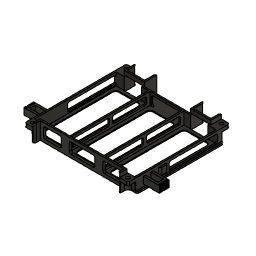
BatteryBase (Autodesk Fusion 360 design; units mm, degrees)
Autodesk Fusion 360 part; units mm, degrees
sketch "草图1" plane through (0, 0, 0) normal (0, 0, 1) x (1, 0, 0)
  line L0 (31, 31.5) -> (-31, 31.5)
  line L1 (-32, 30.5) -> (-32, -30.5)
  line L2 (-31, -31.5) -> (31, -31.5)
  line L3 (32, -30.5) -> (32, 30.5)
  line L4 (32, 31.5) -> (-32, -31.5) construction
  line L5 (-32, 31.5) -> (32, -31.5) construction
  arc A0 (-31, 31.5) -> (-32, 30.5) centre (-31, 30.5) ccw
  arc A1 (-32, -30.5) -> (-31, -31.5) centre (-31, -30.5) ccw
  arc A2 (31, -31.5) -> (32, -30.5) centre (31, -30.5) ccw
  arc A3 (32, 30.5) -> (31, 31.5) centre (31, 30.5) ccw
  dimension "d3" = 1
  dimension "d4" = 1
  dimension "d5" = 1
  dimension "d6" = 1
  dimension "d7" = 64
  dimension "d8" = 63
  constraint horizontal L0
  constraint perpendicular L0 L1
  constraint parallel L0 L2
  constraint parallel L1 L3
  constraint coincident L4 origin
  constraint coincident L5 origin
  constraint coincident L5.start L1
  constraint coincident L5.start L0
  constraint tangent L1 A0
  constraint tangent L0 A0
  constraint coincident L4.end L1
  constraint coincident L4.end L2
  constraint tangent L1 A1
  constraint tangent L2 A1
  constraint coincident L5.end L2
  constraint coincident L5.end L3
  constraint tangent L2 A2
  constraint tangent L3 A2
  constraint coincident L4.start L0
  constraint coincident L4.start L3
  constraint tangent L0 A3
  constraint tangent L3 A3
  measures "d3" radius of A0
  measures "d4" radius of A1
  measures "d5" radius of A2
  measures "d6" radius of A3
  measures "d7" distance of L1 L3
  measures "d8" distance of L0 L2
extrude "拉伸1" add sketch "草图1" along normal blind 10.6 makes body 1
sketch "草图2" plane through (0, 0, 10.6) normal (0, 0, 1) x (-1, 0, 0)
  arc A0 (-32, -30.5) -> (-31, -31.5) centre (-31, -30.5) ccw
  line L0 (-31, -31.5) -> (31, -31.5)
  arc A1 (31, -31.5) -> (32, -30.5) centre (31, -30.5) ccw
  line L1 (32, -30.5) -> (32, 30.5)
  arc A2 (32, 30.5) -> (31, 31.5) centre (31, 30.5) ccw
  line L2 (31, 31.5) -> (-31, 31.5)
  arc A3 (-31, 31.5) -> (-32, 30.5) centre (-31, 30.5) ccw
  line L3 (-32, 30.5) -> (-32, -30.5)
  line L4 (32.1, -24.5) -> (26.9, -24.5)
  line L5 (26.9, -24.5) -> (26.9, -31.5)
  line L6 (26.9, -31.5) -> (32.1, -31.5)
  line L7 (32.1, -31.5) -> (32.1, -24.5)
  line L8 (0, -35) -> (0, 35) construction
  line L9 (42, 0) -> (-42, 0) construction
  line L10 (-26.9, -24.5) -> (-26.9, -31.5)
  line L11 (-26.9, -31.5) -> (-32.1, -31.5)
  line L12 (-32.1, -24.5) -> (-26.9, -24.5)
  line L13 (-32.1, -31.5) -> (-32.1, -24.5)
  line L14 (26.9, 24.5) -> (26.9, 31.5)
  line L15 (26.9, 31.5) -> (32.1, 31.5)
  line L16 (32.1, 31.5) -> (32.1, 24.5)
  line L17 (32.1, 24.5) -> (26.9, 24.5)
  line L18 (-26.9, 31.5) -> (-32.1, 31.5)
  line L19 (-26.9, 24.5) -> (-26.9, 31.5)
  line L20 (-32.1, 24.5) -> (-26.9, 24.5)
  line L21 (-32.1, 31.5) -> (-32.1, 24.5)
  point P0 (-31, -30.5)
  point P1 (-31, -31.5)
  point P2 (31, 30.5)
  point P3 (31, 31.5)
  point P4 (-31, 30.5)
  point P5 (-31, 31.5)
  point P6 (-31, 30.5)
  point P7 (-31, 31.5)
  dimension "d11" = 26.9
  dimension "d12" = 5.2
  dimension "d13" = 7
  constraint horizontal L4
  constraint vertical L5
  constraint horizontal L6
  constraint vertical L7
  constraint coincident L0 L5.end
  constraint perpendicular L2 L8
  constraint perpendicular L3 L9
  constraint symmetric L0.end L8 P1
  constraint symmetric A1.centre L8 P0
  constraint symmetric L4.start L8 L12.start
  constraint symmetric L4.end L8 L10.start
  constraint symmetric L5.end L8 L10.end
  constraint symmetric L6.end L8 L11.end
  constraint symmetric L0.end L9 P3
  constraint symmetric A1.centre L9 P2
  constraint symmetric L4.start L9 L16.end
  constraint symmetric L4.end L9 L14.start
  constraint symmetric L5.end L9 L14.end
  constraint symmetric L6.end L9 L15.end
  constraint symmetric P1 L9 P7
  constraint symmetric P0 L9 P6
  constraint symmetric L9 P0 P6
  constraint symmetric L9 L11.end L18.end
  constraint symmetric L9 L10.end L18.start
  constraint symmetric L9 P1 P7
  constraint symmetric L9 L10.start L19.start
  constraint symmetric L9 L12.start L20.start
  measures "d11" distance of origin L5
  measures "d12" distance of L4.start L4.end
  measures "d13" distance of L4 L6
extrude "拉伸2" cut sketch "草图2" against normal blind 2.5 contours A0 L0 L3 L10 L11 L12 | A0 L3 L11 L12 L13 | A3 L3 L18 L20 L21 | L2 A3 L3 L18 L19 L20 | L0 A1 L1 L4 L5 L6 | A1 L1 L4 L6 L7 | L1 A2 L2 L14 L15 L17 | L1 A2 L15 L16 L17 bodies 1
sketch "草图3" plane through (0, 0, 10.6) normal (0, 0, 1) x (-1, 0, 0)
  line L0 (32, -25) -> (-32, -25)
  line L1 (-32, -25) -> (-32, 27)
  line L2 (-32, 27) -> (32, 27)
  line L3 (32, 27) -> (32, -25)
  dimension "d206" = 25
  dimension "d207" = 32
  dimension "d208" = 32
  dimension "d209" = 27
  constraint horizontal L0
  constraint vertical L1
  constraint horizontal L2
  constraint vertical L3
  measures "d206" distance of origin L0
  measures "d207" distance of origin L3
  measures "d208" distance of origin L1
  measures "d209" distance of origin L2
extrude "拉伸3" cut sketch "草图3" against normal blind 2.5 bodies 1
sketch "草图5" plane through (0, 0, 8.1) normal (0, 0, 1) x (-1, 0, 0)
  circle A0 centre (29.5, -29) radius 1.1
  line L0 (0, -32.9404) -> (0, 32.0596) construction
  line L1 (41.6677, 0) -> (-40.3323, 0) construction
  circle A1 centre (-29.5, -29) radius 1.1
  circle A2 centre (29.5, 29) radius 1.1
  circle A3 centre (-29.5, 29) radius 1.1
  arc A4 (-31, 31.5) -> (-32, 30.5) centre (-31, 30.5) ccw
  line L2 (-32, 30.5) -> (-32, -30.5)
  line L3 (-26.9, 27) -> (-26.9, 31.5)
  line L4 (-26.9, 31.5) -> (-31, 31.5)
  line L5 (32, -30.5) -> (32, 30.5)
  arc A5 (32, 30.5) -> (31, 31.5) centre (31, 30.5) ccw
  line L6 (26.9, 31.5) -> (26.9, 27)
  line L7 (-26.9, -25) -> (26.9, -25)
  line L8 (31, 31.5) -> (26.9, 31.5)
  line L9 (26.9, 27) -> (-26.9, 27)
  arc A6 (-32, -30.5) -> (-31, -31.5) centre (-31, -30.5) ccw
  line L10 (-31, -31.5) -> (-26.9, -31.5)
  line L11 (-26.9, -31.5) -> (-26.9, -25)
  line L12 (26.9, -25) -> (26.9, -31.5)
  line L13 (26.9, -31.5) -> (31, -31.5)
  arc A7 (31, -31.5) -> (32, -30.5) centre (31, -30.5) ccw
  line L14 (31, -31.5) -> (26.9, -31.5)
  line L15 (-26.9, -31.5) -> (-31, -31.5)
  dimension "d20" = 2.2
  dimension "d21" = 29.5
  constraint horizontal L1
  constraint symmetric A0 L0 A1
  constraint symmetric A0 L1 A2
  constraint symmetric L1 A1 A3
  constraint coincident origin L1
  measures "d20" diameter of A0
  measures "d21" distance of A0.centre L0
extrude "拉伸4" cut sketch "草图5" against normal blind 12 contours A0 | A1 | A2 | A3 bodies 1
sketch "草图6" plane through (0, 0, 8.1) normal (0, 0, 1) x (-1, 0, 0)
  line L0 (10, 26.5) -> (-10, 26.5)
  line L1 (-10, 26.5) -> (-10, -24.1)
  line L2 (-10, -24.1) -> (10, -24.1)
  line L3 (10, -24.1) -> (10, 26.5)
  line L4 (11, 26.5) -> (11, -24.1)
  line L5 (11, -24.1) -> (31, -24.1)
  line L6 (31, -24.1) -> (31, 26.5)
  line L7 (31, 26.5) -> (11, 26.5)
  line L8 (-11, -24.1) -> (-11, 26.5)
  line L9 (-31, -24.1) -> (-11, -24.1)
  line L10 (-31, 26.5) -> (-31, -24.1)
  line L11 (-11, 26.5) -> (-31, 26.5)
  point P0 (23, 0)
  dimension "d25" = 50.6
  dimension "d26" = 20
  dimension "d28" = 10
  dimension "d160" = 24.1
  dimension "d200" = 21
  dimension "d201" = 0
  dimension "d204" = -21
  dimension "d205" = 0
  constraint horizontal L0
  constraint vertical L1
  constraint horizontal L2
  constraint vertical L3
  measures "d25" distance of L0 L2
  measures "d26" distance of L1 L3
  measures "d28" distance of origin L3
  measures "d160" distance of origin L2
extrude "拉伸5" cut sketch "草图6" against normal blind 7.5 bodies 1
sketch "草图7" plane through (0, 0, 10.6) normal (0, 0, 1) x (-1, 0, 0)
  line L0 (14.2, -32.5) -> (-14.2, -32.5)
  line L1 (-14.2, -32.5) -> (-14.2, -25)
  line L2 (-14.2, -25) -> (14.2, -25)
  line L3 (14.2, -25) -> (14.2, -32.5)
  line L4 (-26.9, -31.5) -> (26.9, -31.5)
  dimension "d210" = 28.4
  dimension "d211" = 14.2
  dimension "d212" = 7.5
  dimension "d213" = 1
  constraint horizontal L0
  constraint vertical L1
  constraint horizontal L2
  constraint vertical L3
  measures "d210" distance of L0.start L0.end
  measures "d211" distance of origin L3
  measures "d212" distance of L0 L2
  measures "d213" distance of L0 L4
extrude "拉伸6" cut sketch "草图7" against normal blind 10 contours L1 L2 L3 L4 bodies 1
sketch "草图8" plane through (0, 0, 0) normal (0, 0, -1) x (1, 0, 0)
  circle A0 centre (29.5, -29) radius 1.1
  circle A1 centre (29.5, 29) radius 1.1
  circle A2 centre (-29.5, -29) radius 1.1
  circle A3 centre (-29.5, 29) radius 1.1
  arc A4 (31, -31.5) -> (32, -30.5) centre (31, -30.5) ccw
  line L0 (32, -30.5) -> (32, 30.5)
  arc A5 (32, 30.5) -> (31, 31.5) centre (31, 30.5) ccw
  line L1 (31, 31.5) -> (-31, 31.5)
  arc A6 (-31, 31.5) -> (-32, 30.5) centre (-31, 30.5) ccw
  line L2 (-32, 30.5) -> (-32, -30.5)
  arc A7 (-32, -30.5) -> (-31, -31.5) centre (-31, -30.5) ccw
  line L3 (-31, -31.5) -> (31, -31.5)
  line L4 (-27.25, -31.5) -> (-27.25, -29)
  arc A8 (-27.25, -29) -> (-29.5, -26.75) centre (-29.5, -29) ccw
  line L5 (-29.5, -26.75) -> (-32, -26.75)
  line L6 (-27.25, -31.5) -> (-32, -31.5)
  line L7 (-32, -31.5) -> (-32, -26.75)
  line L8 (0, 0) -> (0, -35.7706) construction
  line L9 (27.25, -31.5) -> (32, -31.5)
  line L10 (32, -31.5) -> (32, -26.75)
  circle A9 centre (29.5, -29) radius 1.1
  arc A10 (31, -31.5) -> (32, -30.5) centre (31, -30.5) ccw
  line L11 (27.25, -31.5) -> (27.25, -29)
  line L12 (29.5, -26.75) -> (32, -26.75)
  arc A11 (29.5, -26.75) -> (27.25, -29) centre (29.5, -29) ccw
  line L13 (0, 0) -> (-39, 0) construction
  arc A12 (27.25, 29) -> (29.5, 26.75) centre (29.5, 29) ccw
  line L14 (27.25, 31.5) -> (32, 31.5)
  line L15 (27.25, 31.5) -> (27.25, 29)
  circle A13 centre (29.5, 29) radius 1.1
  arc A14 (32, 30.5) -> (31, 31.5) centre (31, 30.5) ccw
  line L16 (32, 31.5) -> (32, 26.75)
  arc A15 (32, 30.5) -> (31, 31.5) centre (31, 30.5) ccw
  line L17 (29.5, 26.75) -> (32, 26.75)
  circle A16 centre (29.5, 29) radius 1.1
  line L18 (-27.25, 31.5) -> (-32, 31.5)
  line L19 (-32, 31.5) -> (-32, 26.75)
  circle A17 centre (-29.5, 29) radius 1.1
  arc A18 (-31, 31.5) -> (-32, 30.5) centre (-31, 30.5) ccw
  line L20 (-29.5, 26.75) -> (-32, 26.75)
  line L21 (-27.25, 31.5) -> (-27.25, 29)
  arc A19 (-29.5, 26.75) -> (-27.25, 29) centre (-29.5, 29) ccw
  dimension "d260" = 2.25
  constraint coincident L3 L4.start
  constraint perpendicular L3 L4
  constraint coincident A2.centre A8.centre
  constraint coincident L2 L5.end
  constraint horizontal L5
  constraint tangent L4 A8
  constraint tangent A8 L5
  constraint perpendicular L4 L6
  constraint vertical L7
  constraint coincident L8.start L13.start
  constraint perpendicular L3 L8
  constraint symmetric A2 L8 A9
  constraint symmetric L2.end L8 A4.end
  constraint symmetric A7.end L8 A4.start
  constraint symmetric A7 L8 A10
  constraint symmetric L4.start L8 L9.start
  constraint symmetric L4.end L8 L11.end
  constraint symmetric A8.end L8 L12.start
  constraint symmetric A8 L8 A11
  constraint symmetric L5.end L8 L10.end
  constraint symmetric L6.end L8 L9.end
  constraint perpendicular L2 L13
  constraint symmetric A0 L13 A16
  constraint symmetric A2 L13 A17
  constraint symmetric A4.start L13 A5.end
  constraint symmetric A4.end L13 L0.end
  constraint symmetric A4 L13 A14
  constraint symmetric L2.end L13 A6.end
  constraint symmetric A7.end L13 L1.end
  constraint symmetric A7 L13 A18
  constraint symmetric L4.start L13 L18.start
  constraint symmetric L4.end L13 L21.end
  constraint symmetric A8.end L13 L20.start
  constraint symmetric A8 L13 A19
  constraint symmetric L5.end L13 L19.end
  constraint symmetric L6.end L13 L18.end
  constraint symmetric L10.end L13 L16.end
  constraint symmetric L12.start L13 A12.end
  constraint symmetric L9.start L13 L14.start
  constraint symmetric L11.end L13 A12.start
  constraint symmetric L9.end L13 L14.end
  constraint symmetric A9 L13 A13
  constraint symmetric A10 L13 A15
  constraint symmetric A11 L13 A12
  measures "d260" distance of A2.centre L5
extrude "拉伸7" cut sketch "草图8" against normal blind 6 contours A0 A9 | A1 A13 A16 | A3 A17 | A4 L0 L3 L9 L10 A10 L11 L12 A11 | L2 A7 L3 L4 A8 L5 L6 L7 | L0 A5 L1 A12 L14 L15 A14 L16 A15 L17 | L1 A6 L2 L18 L19 A18 L20 L21 A19 bodies 1
sketch "草图9" plane through (0, 0, 10.6) normal (0, 0, 1) x (-1, 0, 0)
  line L0 (14.2, -31.5) -> (26.9, -31.5)
  line L1 (26.9, -31.5) -> (26.9, -25)
  line L2 (25.9, -31.5) -> (15.2, -31.5)
  line L3 (15.2, -31.5) -> (15.2, -26)
  line L4 (15.2, -26) -> (25.9, -26)
  line L5 (25.9, -26) -> (25.9, -31.5)
  line L6 (0, -33) -> (0, 32.4945) construction
  line L7 (-25.9, -31.5) -> (-15.2, -31.5)
  line L8 (-15.2, -26) -> (-25.9, -26)
  line L9 (-25.9, -26) -> (-25.9, -31.5)
  line L10 (-15.2, -31.5) -> (-15.2, -26)
  line L11 (14.2, -25) -> (14.2, -31.5)
  line L12 (26.9, -25) -> (14.2, -25)
  dimension "d49" = 1
  dimension "d216" = 1
  dimension "d217" = 1
  constraint horizontal L2
  constraint vertical L3
  constraint horizontal L4
  constraint vertical L5
  constraint coincident L0 L2.start
  constraint vertical L6
  constraint symmetric L2.start L6 L7.start
  constraint symmetric L2.end L6 L7.end
  constraint symmetric L3.end L6 L8.start
  constraint symmetric L4.end L6 L8.end
  measures "d49" distance of L1 L5
  measures "d216" distance of L4 L12
  measures "d217" distance of L3 L11
extrude "拉伸8" cut sketch "草图9" against normal blind 19 contours L0 L2 L3 L4 L5 | L7 L8 L9 L10 bodies 1
sketch "草图10" plane through (0, 0, 10.6) normal (0, 0, 1) x (-1, 0, 0)
  line L0 (26.9, 27) -> (26.9, 31.5)
  line L1 (26.9, 31.5) -> (-26.9, 31.5)
  line L2 (-26.9, 31.5) -> (-26.9, 27)
  line L3 (25.9, 31.5) -> (-25.9, 31.5)
  line L4 (-25.9, 31.5) -> (-25.9, 28)
  line L5 (-25.9, 28) -> (25.9, 28)
  line L6 (25.9, 28) -> (25.9, 31.5)
  line L7 (-26.9, 27) -> (26.9, 27)
  dimension "d54" = 1
  dimension "d55" = 1
  dimension "d215" = 1
  constraint horizontal L3
  constraint vertical L4
  constraint horizontal L5
  constraint vertical L6
  constraint coincident L1 L3.start
  measures "d54" distance of L0 L6
  measures "d55" distance of L2 L4
  measures "d215" distance of L5 L7
extrude "拉伸9" cut sketch "草图10" against normal blind 19 contours L1 L3 L4 L5 L6 bodies 1
sketch "草图20" plane through (0, 31.5, 0) normal (0, 1, 0) x (-1, 0, 0)
  line L0 (15.2, 0) -> (15.2, 10.6)
  line L1 (15.2, 10.6) -> (14.2, 10.6)
  line L2 (14.2, 10.6) -> (14.2, 0.6)
  line L3 (14.2, 0.6) -> (-14.2, 0.6)
  line L4 (-14.2, 0.6) -> (-14.2, 10.6)
  line L5 (-14.2, 10.6) -> (-15.2, 10.6)
  line L6 (-15.2, 10.6) -> (-15.2, 0)
  line L7 (-15.2, 0) -> (15.2, 0)
extrude "拉伸18" add sketch "草图20" along normal blind 1 bodies 1
sketch "草图12" plane through (0, 0, 0.6) normal (0, 0, 1) x (-1, 0, 0)
  line L0 (6, -22.1) -> (-6, -22.1)
  line L1 (-8, -20.1) -> (-8, 22.5)
  line L2 (-6, 24.5) -> (6, 24.5)
  line L3 (8, 22.5) -> (8, -20.1)
  line L4 (10, -24.1) -> (-10, -24.1)
  line L5 (10, 26.5) -> (10, -24.1)
  line L6 (-10, -24.1) -> (-10, 26.5)
  arc A0 (6, -22.1) -> (8, -20.1) centre (6, -20.1) ccw
  arc A1 (-8, -20.1) -> (-6, -22.1) centre (-6, -20.1) ccw
  arc A2 (8, 22.5) -> (6, 24.5) centre (6, 22.5) ccw
  arc A3 (-6, 24.5) -> (-8, 22.5) centre (-6, 22.5) ccw
  line L7 (27.2, -22.1) -> (15.2, -22.1)
  arc A4 (27.2, -22.1) -> (29.2, -20.1) centre (27.2, -20.1) ccw
  line L8 (29.2, 22.5) -> (29.2, -20.1)
  arc A5 (29.2, 22.5) -> (27.2, 24.5) centre (27.2, 22.5) ccw
  line L9 (15.2, 24.5) -> (27.2, 24.5)
  arc A6 (15.2, 24.5) -> (13.2, 22.5) centre (15.2, 22.5) ccw
  line L10 (13.2, -20.1) -> (13.2, 22.5)
  arc A7 (13.2, -20.1) -> (15.2, -22.1) centre (15.2, -20.1) ccw
  line L11 (-15.2, -22.1) -> (-27.2, -22.1)
  arc A8 (-15.2, -22.1) -> (-13.2, -20.1) centre (-15.2, -20.1) ccw
  line L12 (-13.2, 22.5) -> (-13.2, -20.1)
  arc A9 (-13.2, 22.5) -> (-15.2, 24.5) centre (-15.2, 22.5) ccw
  line L13 (-27.2, 24.5) -> (-15.2, 24.5)
  arc A10 (-27.2, 24.5) -> (-29.2, 22.5) centre (-27.2, 22.5) ccw
  line L14 (-29.2, -20.1) -> (-29.2, 22.5)
  arc A11 (-29.2, -20.1) -> (-27.2, -22.1) centre (-27.2, -20.1) ccw
  line L15 (-26.9, 27) -> (26.9, 27)
  dimension "d172" = 2
  dimension "d173" = 2
  dimension "d174" = 2
  dimension "d175" = 2
  dimension "d178" = 21.2
  dimension "d179" = 0
  dimension "d182" = -21.2
  dimension "d183" = 0
  dimension "d222" = 2.5
  constraint horizontal L0
  constraint vertical L1
  constraint horizontal L2
  constraint vertical L3
  constraint tangent L0 A0
  constraint tangent L3 A0
  constraint tangent L0 A1
  constraint tangent L1 A1
  constraint equal A0 A1
  constraint tangent L2 A2
  constraint tangent L3 A2
  constraint equal A0 A2
  constraint tangent L1 A3
  constraint tangent L2 A3
  constraint equal A0 A3
  measures "d172" distance of L0 L4
  measures "d173" distance of L3 L5
  measures "d174" distance of L1 L6
  measures "d175" radius of A0
  measures "d222" distance of L2 L15
extrude "拉伸11" cut sketch "草图12" against normal blind 3 bodies 1
sketch "草图22" plane through (-32, 0, 0) normal (-1, 0, 0) x (0, -1, 0)
  line L0 (30.5, 8.1) -> (-30.5, 8.1)
  line L1 (-30.5, 8.1) -> (-30.5, 6)
  line L2 (-26.75, 0) -> (26.75, 0)
  line L3 (30.5, 6) -> (30.5, 8.1)
  line L4 (-26.75, 0) -> (26.75, 0)
  line L5 (26.75, 0) -> (26.75, 1)
  line L6 (26.75, 1) -> (-26.75, 1)
  line L7 (-26.75, 1) -> (-26.75, 0)
  line L8 (-26.75, 6) -> (-26.75, 0)
  line L9 (26.75, 0) -> (26.75, 6)
  line L10 (26.75, 6) -> (30.5, 6)
  line L11 (-30.5, 6) -> (-26.75, 6)
  dimension "d229" = 1
  dimension "d230" = 3.75
  dimension "d231" = 3.75
  constraint horizontal L4
  constraint vertical L5
  constraint horizontal L6
  constraint vertical L7
  constraint coincident L2 L4.start
  measures "d229" distance of L4 L6
  measures "d230" distance of L1 L7
  measures "d231" distance of L3 L5
extrude "拉伸20" add sketch "草图22" along normal blind 1 separate body contours L2 L4 L5 L6 L7 L8 L9 makes body 2
mirror "镜像3" about plane through (0, 0, 0) normal (1, 0, 0) of "拉伸20" makes body 3
fillet "圆角11" radius 1 2 edges at (-33, -26.75, 0.5) (-33, 26.75, 0.5) on bodies 2 3
fillet "圆角11" radius 1 2 edges at (33, -26.75, 0.5) (33, 26.75, 0.5) on bodies 2 3
sketch "草图17" plane through (-32, 0, 0) normal (-1, 0, 0) x (0, -1, 0)
  line L0 (30.5, 6) -> (30.5, 8.1)
  line L1 (-30.5, 8.1) -> (-30.5, 6)
  line L2 (16, 6.6) -> (22, 6.6)
  line L3 (22, 6.6) -> (22, 2.5)
  line L4 (22, 2.5) -> (16, 2.5)
  line L5 (16, 2.5) -> (16, 6.6)
  line L6 (30.5, 8.1) -> (-30.5, 8.1)
  line L7 (-26.75, 0) -> (26.75, 0)
  line L8 (-26.75, 6) -> (-26.75, 0)
  line L9 (26.75, 0) -> (26.75, 6)
  line L10 (26.75, 6) -> (30.5, 6)
  line L11 (-30.5, 6) -> (-26.75, 6)
  dimension "d151" = 6
  dimension "d152" = 16
  dimension "d218" = 1.5
  dimension "d261" = 2.5
  constraint horizontal L2
  constraint vertical L3
  constraint horizontal L4
  constraint vertical L5
  measures "d151" distance of L3 L5
  measures "d152" distance of origin L5
  measures "d218" distance of L2 L6
  measures "d261" distance of L4 L7
extrude "拉伸15" add sketch "草图17" along normal blind 9 separate body contours L2 L3 L4 L5 makes body 4
sketch "草图19" plane through (0, 0, 6.6) normal (0, 0, 1) x (-1, 0, 0)
  line L0 (32, 22) -> (32, 16)
  line L1 (32, 16) -> (41, 16)
  line L2 (41, 16) -> (41, 22)
  line L3 (41, 22) -> (32, 22)
  line L4 (39.7, 17.3) -> (32, 17.3)
  line L5 (32, 17.3) -> (32, 20.7)
  line L6 (32, 20.7) -> (39.7, 20.7)
  line L7 (39.7, 20.7) -> (39.7, 17.3)
  line L8 (0, -35) -> (0, 35) construction
  line L9 (-39.7, 17.3) -> (-32, 17.3)
  line L10 (-39.7, 20.7) -> (-39.7, 17.3)
  line L11 (-32, 20.7) -> (-39.7, 20.7)
  line L12 (-32, 17.3) -> (-32, 20.7)
  dimension "d192" = 1.3
  dimension "d193" = 1.3
  dimension "d194" = 1.3
  constraint horizontal L4
  constraint vertical L5
  constraint horizontal L6
  constraint vertical L7
  constraint collinear L0 L5
  constraint vertical L8
  constraint symmetric L4.start L8 L9.start
  constraint symmetric L4.end L8 L9.end
  constraint symmetric L5.end L8 L11.start
  constraint symmetric L6.end L8 L10.start
  measures "d192" distance of L1 L4
  measures "d193" distance of L2 L7
  measures "d194" distance of L3 L6
sketch "草图18" plane through (-41, 0, 0) normal (-1, 0, 0) x (0, -1, 0)
  line L0 (16, 2.5) -> (22, 2.5)
  line L1 (22, 2.5) -> (22, 6.6)
  line L2 (22, 6.6) -> (16, 6.6)
  line L3 (16, 6.6) -> (16, 2.5)
  line L4 (16, 6.6) -> (16.5, 6.6)
  line L5 (16.5, 6.6) -> (16.5, 2.5)
  line L6 (16.5, 2.5) -> (16, 2.5)
  line L7 (16, 2.5) -> (16, 6.6)
  line L8 (17.4167, 6.6) -> (17.4167, 2.5)
  line L9 (16.9167, 6.6) -> (16.9167, 2.5)
  line L10 (17.4167, 2.5) -> (16.9167, 2.5)
  line L11 (16.9167, 2.5) -> (16.9167, 6.6)
  line L12 (16.9167, 6.6) -> (17.4167, 6.6)
  line L13 (18.3333, 6.6) -> (18.3333, 2.5)
  line L14 (17.8333, 6.6) -> (17.8333, 2.5)
  line L15 (18.3333, 2.5) -> (17.8333, 2.5)
  line L16 (17.8333, 2.5) -> (17.8333, 6.6)
  line L17 (17.8333, 6.6) -> (18.3333, 6.6)
  line L18 (19.25, 6.6) -> (19.25, 2.5)
  line L19 (18.75, 6.6) -> (18.75, 2.5)
  line L20 (19.25, 2.5) -> (18.75, 2.5)
  line L21 (18.75, 2.5) -> (18.75, 6.6)
  line L22 (18.75, 6.6) -> (19.25, 6.6)
  line L23 (20.1667, 6.6) -> (20.1667, 2.5)
  line L24 (19.6667, 6.6) -> (19.6667, 2.5)
  line L25 (20.1667, 2.5) -> (19.6667, 2.5)
  line L26 (19.6667, 2.5) -> (19.6667, 6.6)
  line L27 (19.6667, 6.6) -> (20.1667, 6.6)
  line L28 (21.0833, 6.6) -> (21.0833, 2.5)
  line L29 (20.5833, 6.6) -> (20.5833, 2.5)
  line L30 (21.0833, 2.5) -> (20.5833, 2.5)
  line L31 (20.5833, 2.5) -> (20.5833, 6.6)
  line L32 (20.5833, 6.6) -> (21.0833, 6.6)
  line L33 (22, 6.6) -> (22, 2.5)
  line L34 (21.5, 6.6) -> (21.5, 2.5)
  line L35 (22, 2.5) -> (21.5, 2.5)
  line L36 (21.5, 2.5) -> (21.5, 6.6)
  line L37 (21.5, 6.6) -> (22, 6.6)
  dimension "d153" = 0.5
  dimension "d156" = 5.5
  dimension "d157" = 0
  constraint horizontal L4
  constraint vertical L5
  constraint horizontal L6
  constraint vertical L7
  constraint coincident L0 L5.end
  constraint coincident L2.end L3.start
  measures "d153" distance of L5 L7
extrude "拉伸16" add sketch "草图18" along normal blind 1 contours L0 L2 L3 L4 L5 L6 L7 | L0 L2 L8 L9 L10 L11 L12 | L0 L2 L13 L14 L15 L16 L17 | L0 L2 L18 L19 L20 L21 L22 | L0 L2 L23 L24 L25 L26 L27 | L0 L2 L28 L29 L30 L31 L32 | L0 L1 L2 L33 L34 L35 L36 L37 bodies 4
mirror "镜像1" about plane through (0, 0, 0) normal (1, 0, 0) of bodies 4 makes body 5
extrude "拉伸17" cut sketch "草图19" against normal blind 8 contours L0 L4 L5 L6 L7 | L9 L10 L11 L12 bodies 4 5
sketch "草图15" plane through (-32, 0, 0) normal (-1, 0, 0) x (0, -1, 0)
  line L0 (-26.75, 0) -> (26.75, 0)
  line L1 (30.5, 6) -> (30.5, 8.1)
  line L2 (-30.5, 8.1) -> (-30.5, 6)
  line L3 (7.5, 6.6) -> (12.5, 6.6)
  line L4 (12.5, 6.6) -> (12.5, 2.5)
  line L5 (12.5, 2.5) -> (7.5, 2.5)
  line L6 (7.5, 2.5) -> (7.5, 6.6)
  line L7 (30.5, 8.1) -> (-30.5, 8.1)
  line L8 (-26.75, 6) -> (-26.75, 0)
  line L9 (26.75, 0) -> (26.75, 6)
  line L10 (26.75, 6) -> (30.5, 6)
  line L11 (-30.5, 6) -> (-26.75, 6)
  dimension "d188" = 7.5
  dimension "d189" = 5
  dimension "d191" = 2.5
  dimension "d219" = 1.5
  constraint horizontal L3
  constraint vertical L4
  constraint horizontal L5
  constraint vertical L6
  measures "d188" distance of origin L6
  measures "d189" distance of L4 L6
  measures "d191" distance of L0 L5
  measures "d219" distance of L3 L7
extrude "拉伸14" add sketch "草图15" along normal blind 1 separate body contours L3 L4 L5 L6 makes body 6
chamfer "倒角2" distance 1 distance2 1 1 edges at (-33, -7.5, 4.55) measured on face at (-33, -9.1667, 5.2333) on bodies 6
chamfer "倒角2" distance 1 distance2 1 1 edges at (-33, -12.5, 4.55) measured on face at (-33, -9.1667, 5.2333) on bodies 6
mirror "镜像2" about plane through (0, 0, 0) normal (1, 0, 0) of bodies 6 makes body 7
sketch "草图23" plane through (-11, 0, 0) normal (-1, 0, 0) x (0, -1, 0)
  line L0 (26.5, 8.1) -> (-24.1, 8.1)
  line L1 (-24.1, 8.1) -> (-24.1, 0.6)
  line L2 (26.5, 0.6) -> (26.5, 8.1)
  line L3 (-21.1, 6.6) -> (-2, 6.6)
  line L4 (-1, 5.6) -> (-1, 3.1)
  line L5 (-2, 2.1) -> (-21.1, 2.1)
  line L6 (-22.1, 3.1) -> (-22.1, 5.6)
  line L7 (2, 6.6) -> (23.5, 6.6)
  line L8 (24.5, 5.6) -> (24.5, 3.1)
  line L9 (23.5, 2.1) -> (2, 2.1)
  line L10 (1, 3.1) -> (1, 5.6)
  arc A0 (-21.1, 6.6) -> (-22.1, 5.6) centre (-21.1, 5.6) ccw
  arc A1 (-22.1, 3.1) -> (-21.1, 2.1) centre (-21.1, 3.1) ccw
  arc A2 (-2, 2.1) -> (-1, 3.1) centre (-2, 3.1) ccw
  arc A3 (-1, 5.6) -> (-2, 6.6) centre (-2, 5.6) ccw
  arc A4 (2, 6.6) -> (1, 5.6) centre (2, 5.6) ccw
  arc A5 (1, 3.1) -> (2, 2.1) centre (2, 3.1) ccw
  arc A6 (23.5, 2.1) -> (24.5, 3.1) centre (23.5, 3.1) ccw
  arc A7 (24.5, 5.6) -> (23.5, 6.6) centre (23.5, 5.6) ccw
  line L11 (-24.1, 0.6) -> (26.5, 0.6)
  dimension "d240" = 1
  dimension "d241" = 2
  dimension "d242" = 1.5
  dimension "d244" = 1
  dimension "d245" = 1
  dimension "d246" = 1
  dimension "d247" = 1.5
  dimension "d249" = 2
  constraint horizontal L3
  constraint vertical L4
  constraint horizontal L5
  constraint vertical L6
  constraint horizontal L7
  constraint vertical L8
  constraint horizontal L9
  constraint vertical L10
  constraint tangent L3 A0
  constraint tangent L6 A0
  constraint tangent L5 A1
  constraint tangent L6 A1
  constraint equal A0 A1
  constraint tangent L4 A2
  constraint tangent L5 A2
  constraint equal A0 A2
  constraint tangent L3 A3
  constraint tangent L4 A3
  constraint equal A0 A3
  constraint tangent L7 A4
  constraint tangent L10 A4
  constraint tangent L9 A5
  constraint tangent L10 A5
  constraint equal A4 A5
  constraint tangent L8 A6
  constraint tangent L9 A6
  constraint equal A4 A6
  constraint tangent L7 A7
  constraint tangent L8 A7
  constraint equal A4 A7
  measures "d240" radius of A0
  measures "d241" distance of L1 L6
  measures "d242" distance of L0 L3
  measures "d244" distance of origin L4
  measures "d245" radius of A4
  measures "d246" distance of origin L10
  measures "d247" distance of L0 L7
  measures "d249" distance of L2 L8
extrude "拉伸21" cut sketch "草图23" against normal blind 22 contours L3 L4 L5 L6 A0 A1 A2 A3 | L7 L8 L9 L10 A4 A5 A6 A7 bodies 1
sketch "草图24" plane through (31, 0, 0) normal (-1, 0, 0) x (0, -1, 0)
  line L0 (26.5, 8.1) -> (-24.1, 8.1)
  line L1 (-24.1, 8.1) -> (-24.1, 0.6)
  line L2 (26.5, 0.6) -> (26.5, 8.1)
  line L3 (-23.1, 6.6) -> (4.9, 6.6)
  line L4 (5.9, 5.6) -> (5.9, 2.2)
  line L5 (4.9, 1.2) -> (-23.1, 1.2)
  line L6 (-24.1, 2.2) -> (-24.1, 5.6)
  arc A0 (-23.1, 6.6) -> (-24.1, 5.6) centre (-23.1, 5.6) ccw
  arc A1 (-24.1, 2.2) -> (-23.1, 1.2) centre (-23.1, 2.2) ccw
  arc A2 (4.9, 1.2) -> (5.9, 2.2) centre (4.9, 2.2) ccw
  arc A3 (5.9, 5.6) -> (4.9, 6.6) centre (4.9, 5.6) ccw
  line L7 (-24.1, 0.6) -> (26.5, 0.6)
  dimension "d252" = 1.5
  dimension "d254" = 1
  dimension "d255" = 30
  constraint horizontal L3
  constraint vertical L4
  constraint horizontal L5
  constraint vertical L6
  constraint tangent L3 A0
  constraint tangent L6 A0
  constraint tangent L5 A1
  constraint tangent L6 A1
  constraint equal A0 A1
  constraint tangent L4 A2
  constraint tangent L5 A2
  constraint equal A0 A2
  constraint tangent L3 A3
  constraint tangent L4 A3
  constraint equal A0 A3
  constraint collinear L1 L6
  measures "d252" distance of L0 L3
  measures "d254" radius of A0
  measures "d255" distance of L4 L6
extrude "拉伸22" cut sketch "草图24" against normal blind 1 contours L1 L3 L4 L5 L6 A0 A1 A2 A3 bodies 1
sketch "草图25" plane through (-31, 0, 0) normal (1, 0, 0) x (0, 1, 0)
  line L0 (24.1, 8.1) -> (-26.5, 8.1)
  line L1 (-26.5, 8.1) -> (-26.5, 0.6)
  line L2 (24.1, 0.6) -> (24.1, 8.1)
  arc A0 (-4.9, 6.6) -> (-5.9, 5.6) centre (-4.9, 5.6) ccw
  line L3 (-5.9, 2.2) -> (-5.9, 5.6)
  arc A1 (-5.9, 2.2) -> (-4.9, 1.2) centre (-4.9, 2.2) ccw
  line L4 (23.1, 1.2) -> (-4.9, 1.2)
  arc A2 (23.1, 1.2) -> (24.1, 2.2) centre (23.1, 2.2) ccw
  line L5 (24.1, 5.6) -> (24.1, 2.2)
  arc A3 (24.1, 5.6) -> (23.1, 6.6) centre (23.1, 5.6) ccw
  line L6 (-4.9, 6.6) -> (23.1, 6.6)
  line L7 (-26.5, 0.6) -> (24.1, 0.6)
extrude "拉伸23" cut sketch "草图25" against normal blind 1 contours L2 A0 L3 A1 L4 A2 L5 A3 L6 bodies 1
sketch "草图26" plane through (0, -28, 0) normal (0, -1, 0) x (1, 0, 0)
  line L0 (-25.9, 0) -> (25.9, 0)
  line L1 (25.9, 0) -> (25.9, 10.6)
  line L2 (25.9, 10.6) -> (-25.9, 10.6)
  line L3 (-25.9, 10.6) -> (-25.9, 0)
  line L4 (-6.9, 8.6) -> (6.9, 8.6)
  line L5 (7.9, 7.6) -> (7.9, 3)
  line L6 (6.9, 2) -> (-6.9, 2)
  line L7 (-7.9, 3) -> (-7.9, 7.6)
  arc A0 (-6.9, 8.6) -> (-7.9, 7.6) centre (-6.9, 7.6) ccw
  arc A1 (-7.9, 3) -> (-6.9, 2) centre (-6.9, 3) ccw
  arc A2 (6.9, 2) -> (7.9, 3) centre (6.9, 3) ccw
  arc A3 (7.9, 7.6) -> (6.9, 8.6) centre (6.9, 7.6) ccw
  line L8 (-22.9, 8.6) -> (-13.9, 8.6)
  line L9 (-12.9, 7.6) -> (-12.9, 3)
  line L10 (-13.9, 2) -> (-22.9, 2)
  line L11 (-23.9, 3) -> (-23.9, 7.6)
  arc A4 (-22.9, 8.6) -> (-23.9, 7.6) centre (-22.9, 7.6) ccw
  arc A5 (-23.9, 3) -> (-22.9, 2) centre (-22.9, 3) ccw
  arc A6 (-13.9, 2) -> (-12.9, 3) centre (-13.9, 3) ccw
  arc A7 (-12.9, 7.6) -> (-13.9, 8.6) centre (-13.9, 7.6) ccw
  line L12 (0, 0) -> (0, 13.2372) construction
  arc A8 (12.9, 3) -> (13.9, 2) centre (13.9, 3) ccw
  arc A9 (23.9, 7.6) -> (22.9, 8.6) centre (22.9, 7.6) ccw
  arc A10 (22.9, 2) -> (23.9, 3) centre (22.9, 3) ccw
  line L13 (22.9, 8.6) -> (13.9, 8.6)
  arc A11 (13.9, 8.6) -> (12.9, 7.6) centre (13.9, 7.6) ccw
  line L14 (23.9, 3) -> (23.9, 7.6)
  line L15 (13.9, 2) -> (22.9, 2)
  line L16 (12.9, 7.6) -> (12.9, 3)
  point P0 (25.9, 0)
  dimension "d262" = 1
  dimension "d263" = 2
  dimension "d264" = 18
  dimension "d265" = 18
  dimension "d266" = 2
  dimension "d267" = 1
  dimension "d268" = 2
  dimension "d269" = 5
  dimension "d270" = 2
  dimension "d273" = 2
  constraint horizontal L4
  constraint vertical L5
  constraint horizontal L6
  constraint vertical L7
  constraint tangent L4 A0
  constraint tangent L7 A0
  constraint tangent L6 A1
  constraint tangent L7 A1
  constraint equal A0 A1
  constraint tangent L5 A2
  constraint tangent L6 A2
  constraint equal A0 A2
  constraint tangent L4 A3
  constraint tangent L5 A3
  constraint equal A0 A3
  constraint horizontal L8
  constraint vertical L9
  constraint horizontal L10
  constraint vertical L11
  constraint tangent L8 A4
  constraint tangent L11 A4
  constraint tangent L10 A5
  constraint tangent L11 A5
  constraint equal A4 A5
  constraint tangent L9 A6
  constraint tangent L10 A6
  constraint equal A4 A6
  constraint tangent L8 A7
  constraint tangent L9 A7
  constraint equal A4 A7
  constraint coincident L12.start origin
  constraint perpendicular L2 L12
  constraint symmetric L0.start L12 P0
  constraint symmetric L8.start L12 A9.end
  constraint symmetric L11.end L12 A9.start
  constraint symmetric A4 L12 A9
  constraint symmetric L10.end L12 A10.start
  constraint symmetric L11.start L12 A10.end
  constraint symmetric A5 L12 A10
  constraint symmetric L9.end L12 A8.start
  constraint symmetric L10.start L12 A8.end
  constraint symmetric A6 L12 A8
  constraint symmetric L8.end L12 L13.end
  constraint symmetric L9.start L12 A11.end
  constraint symmetric A7 L12 A11
  measures "d262" radius of A0
  measures "d263" distance of L2 L4
  measures "d264" distance of L1 L5
  measures "d265" distance of L3 L7
  measures "d266" distance of L0 L6
  measures "d267" radius of A4
  measures "d268" distance of L2 L8
  measures "d269" distance of L7 L9
  measures "d270" distance of L0 L10
  measures "d273" distance of L3 L11
extrude "拉伸24" cut sketch "草图26" against normal blind 2 contours L4 L5 L6 L7 A0 A1 A2 A3 | L8 L9 L10 L11 A4 A5 A6 A7 | A8 A9 A10 L13 A11 L14 L15 L16 bodies 1
sketch "草图27" plane through (0, 26, 0) normal (0, 1, 0) x (-1, 0, 0)
  line L0 (15.2, 0) -> (25.9, 0)
  line L1 (25.9, 0) -> (25.9, 10.6)
  line L2 (25.9, 10.6) -> (15.2, 10.6)
  line L3 (15.2, 10.6) -> (15.2, 0)
  line L4 (-15.2, 0) -> (-15.2, 10.6)
  line L5 (-25.9, 10.6) -> (-25.9, 0)
  line L6 (-25.9, 8.1) -> (-15.2, 8.1)
  line L7 (-15.2, 8.1) -> (-15.2, 0)
  line L8 (-15.2, 0) -> (-25.9, 0)
  line L9 (-25.9, 0) -> (-25.9, 8.1)
  line L10 (15.2, 0) -> (25.9, 0)
  line L11 (25.9, 0) -> (25.9, 8.1)
  line L12 (25.9, 8.1) -> (15.2, 8.1)
  line L13 (15.2, 8.1) -> (15.2, 0)
  line L14 (-25.9, 0) -> (-15.2, 0)
  line L15 (-15.2, 10.6) -> (-25.9, 10.6)
  dimension "d275" = 2.5
  constraint horizontal L6
  constraint vertical L7
  constraint horizontal L8
  constraint vertical L9
  constraint coincident L4.start L7.end
  constraint coincident L5 L6.start
  constraint horizontal L10
  constraint vertical L11
  constraint horizontal L12
  constraint vertical L13
  constraint coincident L1 L11.end
  constraint coincident L0.start L3.end
  measures "d275" distance of L2 L12
extrude "拉伸25" cut sketch "草图27" against normal blind 2 contours L0 L1 L3 L10 L11 L12 L13 | L4 L5 L6 L7 L8 L9 L14 bodies 1
sketch "草图28" plane through (0, 25, 0) normal (0, 1, 0) x (-1, 0, 0)
  line L0 (14.2, 8.1) -> (-14.2, 8.1)
  line L1 (-14.2, 8.1) -> (-14.2, 0.6)
  line L2 (-14.2, 0.6) -> (14.2, 0.6)
  line L3 (14.2, 0.6) -> (14.2, 8.1)
  line L4 (-8.2, 0.6) -> (8.2, 0.6)
  line L5 (9.2, 1.6) -> (9.2, 5.6)
  line L6 (8.2, 6.6) -> (-8.2, 6.6)
  line L7 (-9.2, 5.6) -> (-9.2, 1.6)
  arc A0 (-8.2, 6.6) -> (-9.2, 5.6) centre (-8.2, 5.6) ccw
  arc A1 (-9.2, 1.6) -> (-8.2, 0.6) centre (-8.2, 1.6) ccw
  arc A2 (8.2, 0.6) -> (9.2, 1.6) centre (8.2, 1.6) ccw
  arc A3 (9.2, 5.6) -> (8.2, 6.6) centre (8.2, 5.6) ccw
  dimension "d278" = 5
  dimension "d279" = 5
  dimension "d280" = 1.5
  dimension "d281" = 1
  constraint horizontal L4
  constraint vertical L5
  constraint horizontal L6
  constraint vertical L7
  constraint tangent L6 A0
  constraint tangent L7 A0
  constraint tangent L4 A1
  constraint tangent L7 A1
  constraint equal A0 A1
  constraint tangent L4 A2
  constraint tangent L5 A2
  constraint equal A0 A2
  constraint tangent L5 A3
  constraint tangent L6 A3
  constraint equal A0 A3
  constraint collinear L2 L4
  measures "d278" distance of L1 L7
  measures "d279" distance of L3 L5
  measures "d280" distance of L0 L6
  measures "d281" radius of A0
extrude "拉伸26" cut sketch "草图28" against normal blind 1 contours L2 L4 L5 L6 L7 A0 A1 A2 A3 bodies 1
fillet "圆角9" radius 1 2 edges at (25.9, 31.5, 5.3) (-25.9, 31.5, 5.3) on bodies 1
fillet "圆角9" radius 1 2 edges at (-15.2, 32.5, 5.3) (15.2, 32.5, 5.3) on bodies 1
fillet "圆角10" radius 1 2 edges at (-25.9, -31.5, 5.3) (25.9, -31.5, 5.3) on bodies 1
